Autodesk Inventor part; units mm, degrees
(part 2 of 2)
sketch "Sketch20" plane through (6.35, 0, 0) normal (1, 0, 0) x (0, 0, -1)
  line L0 (-19.4443, 227.7716) -> (-198.6709, 407.7544) construction
  line L1 (-19.4443, 227.7716) -> (0, 0) construction
  circle A0 centre (-198.6709, 407.7544) radius 14.2875
  circle A1 centre (-198.6709, 407.7544) radius 25.4 construction
  arc A2 (-180.6726, 425.6771) -> (-216.6692, 389.8318) centre (-198.6709, 407.7544) ccw
  circle A3 centre (0, 0) radius 14.2875 projected
  arc A4 (-50.2264, 149.2557) -> (-54.8964, 147.6019) centre (0, 0) ccw projected
  arc A5 (-59.2639, 135.1204) -> (-53.6386, 137.4505) centre (-57.3822, 138.5329) ccw projected
  arc A6 (-65.5527, 143.188) -> (-70.0243, 141.0551) centre (0, 0) ccw projected
  arc A7 (-73.0632, 128.1854) -> (-67.7123, 131.0907) centre (-71.5485, 131.776) ccw projected
  arc A8 (-80.1608, 135.5514) -> (-84.385, 132.9629) centre (0, 0) ccw projected
  arc A9 (-86.062, 119.846) -> (-81.044, 123.2948) centre (-84.9309, 123.5752) ccw projected
  arc A10 (-93.8907, 126.4298) -> (-97.8211, 123.4139) centre (0, 0) ccw projected
  arc A11 (-98.1178, 110.1936) -> (-93.4879, 114.1479) centre (-97.3828, 114.0206) ccw projected
  arc A12 (-106.5918, 115.9229) -> (-110.1855, 112.5127) centre (0, 0) ccw projected
  arc A13 (-109.0987, 99.3338) -> (-104.9075, 103.7505) centre (-108.7677, 103.2167) ccw projected
  arc A14 (-118.1252, 104.146) -> (-121.3427, 100.3788) centre (0, 0) ccw projected
  arc A15 (-118.8843, 87.3857) -> (-115.1776, 92.2163) centre (-118.9609, 91.2819) ccw projected
  arc A16 (-128.3643, 91.2281) -> (-131.1704, 87.1452) centre (0, 0) ccw projected
  arc A17 (-127.3673, 74.4802) -> (-124.1859, 79.6718) centre (-127.8508, 78.3471) ccw projected
  arc A18 (-137.197, 77.3106) -> (-139.561, 72.9568) centre (0, 0) ccw projected
  arc A19 (-134.4549, 60.7587) -> (-131.8336, 66.2544) centre (-135.3399, 64.5538) ccw projected
  arc A20 (-144.5266, 62.5461) -> (-146.4225, 57.969) centre (0, 0) ccw projected
  arc A21 (-140.0693, 46.3715) -> (-138.0368, 52.1111) centre (-141.3462, 50.0533) ccw projected
  arc A22 (-150.2727, 47.0963) -> (-151.6798, 42.3461) centre (0, 0) ccw projected
  arc A23 (-144.1492, 31.4762) -> (-142.7278, 37.3968) centre (-145.8039, 35.0044) ccw projected
  arc A24 (-154.3724, 31.1305) -> (-155.2752, 26.2593) centre (0, 0) ccw projected
  arc A25 (-146.6497, 16.2361) -> (-145.8549, 22.2728) centre (-148.6641, 19.572) ccw projected
  arc A26 (7.613, -24.2323) -> (25.308, 2.1605) centre (0, 0) ccw projected
  arc A27 (-156.7808, 14.8237) -> (-157.1695, 9.8848) centre (0, 0) ccw projected
  arc A28 (-147.5434, 0.8181) -> (-147.384, 6.9048) centre (-149.8956, 3.9252) ccw projected
  arc A29 (-157.4714, -1.6456) -> (-157.3417, -6.5981) centre (0, 0) ccw projected
  arc A30 (-146.8207, -14.6089) -> (-147.2984, -8.5388) centre (-149.4847, -11.7647) ccw projected
  arc A31 (-156.4367, -18.0968) -> (-155.7901, -23.0086) centre (0, 0) ccw projected
  arc A32 (-144.4893, -29.8758) -> (-145.5989, -23.8889) centre (-147.4361, -27.3257) ccw projected
  arc A33 (-153.6881, -34.3498) -> (-152.5316, -39.1671) centre (0, 0) ccw projected
  arc A34 (-140.575, -44.8154) -> (-142.3043, -38.9773) centre (-143.7721, -42.5872) ccw projected
  arc A35 (-149.2557, -50.2264) -> (-147.6019, -54.8964) centre (0, 0) ccw projected
  arc A36 (-135.1204, -59.2639) -> (-137.4505, -53.6386) centre (-138.5329, -57.3822) ccw projected
  arc A37 (-143.188, -65.5527) -> (-141.0551, -70.0243) centre (0, 0) ccw projected
  arc A38 (-130.9051, -67.7501) -> (-131.0907, -67.7123) centre (-131.776, -71.5485) ccw projected
  line L2 (-130.9051, -67.7501) -> (7.613, -24.2323) projected
  arc A39 (-44.8154, 140.575) -> (-38.9773, 142.3043) centre (-42.5872, 143.7721) ccw projected
  circle A40 centre (-19.4443, 227.7716) radius 14.2875 projected
  line L3 (25.308, 2.1605) -> (5.8637, 229.932) projected
  arc A41 (5.8637, 229.932) -> (-44.787, 226.0661) centre (-19.4443, 227.7716) ccw projected
  line L4 (-44.787, 226.0661) -> (-39.3751, 145.6486) projected
  line L5 (5.8637, 229.932) -> (-44.7522, 225.6111)
  line L6 (5.8637, 229.932) -> (25.308, 2.1605) projected
  line L7 (-39.3751, 145.6486) -> (-44.787, 226.0661) projected
  line L8 (-216.6692, 389.8318) -> (-44.1488, 216.5834)
  line L9 (-180.6726, 425.6771) -> (-1.446, 245.6942)
  arc A42 (5.8637, 229.932) -> (-44.787, 226.0661) centre (-19.4443, 227.7716) ccw projected
  point P0 (-44.1488, 216.5834)
  dimension "d130" = 254
  dimension "d131" = 140
  dimension "d132" = 28.575
  dimension "d133" = 50.8
  dimension "d156" = 0
  constraints: 10 end point, 6 point on circle, 3 centre point, 3 coincident, 3 tangent, 1 concentric, 1 midpoint, 1 point on line, 35 other
  measures "d130" distance of L0.start L0.end
  measures "d131" angle of L1 L0
  measures "d132" diameter of A0
  measures "d133" diameter of A1
  measures "d156" angle of L8 L9
extrude "Extrusion21" add sketch "Sketch20" against normal blind 6.35 contours L9 A41 L4 L8 A2
sketch "Sketch21" plane through (6.35, 0, 0) normal (1, 0, 0) x (0, 0, -1)
  circle A0 centre (0, 0) radius 146.05
  circle A1 centre (0, 0) radius 97.155
  circle A2 centre (0, 0) radius 80.01
  line L0 (0, 0) -> (-128.3643, 91.2281)
  line L1 (0, 0) -> (0, -146.05)
  line L2 (0, 0) -> (-154.3724, 31.1305)
  arc A3 (-127.3673, 74.4802) -> (-124.1859, 79.6718) centre (-127.8508, 78.3471) ccw projected
  point P0 (0, -97.155)
  point P1 (0, -80.01)
  point P2 (-65.2173, 46.3497)
  point P3 (-79.1925, 56.2818)
  point P4 (-78.4311, 15.8163)
  point P5 (-95.2378, 19.2055)
  dimension "d137" = 292.1
  dimension "d138" = 48.895
  dimension "d139" = 17.145
  constraints: 6 end point, 3 coincident, 2 centre point, 1 vertical, 1 vertical alignment, 2 other
  measures "d139" radial gap between concentric circles of A1 A2
extrude "Extrusion22" cut sketch "Sketch21" against normal blind 6.35 contours A1 L2 A2 L1 | A1 L0 A2 L2
fillet "Fillet2" radius 8.5725 2 edges at (3.175, 56.2818, 79.1925) (3.175, 46.3497, 65.2173)
fillet "Fillet3" radius 6.35 2 edges at (3.175, -52.3392, 81.8517) (3.175, -46.9727, 64.7701)
sketch "Sketch22" plane through (0, 0, 0) normal (-1, 0, 0) x (0, 0, 1)
  circle A0 centre (19.4443, 227.7716) radius 14.2875 projected
  circle A1 centre (19.4443, 227.7716) radius 25.4
  circle A2 centre (198.6709, 407.7544) radius 14.2875 projected
  circle A3 centre (198.6709, 407.7544) radius 25.4
  arc A4 (216.6692, 389.8318) -> (44.7712, 225.8313) centre (235.9913, 209.2855) ccw projected
  line L0 (216.6692, 389.8318) -> (37.4426, 209.8489)
  arc A5 (60.2698, -45.5588) -> (67.5328, -42.906) centre (62.173, -39.5007) ccw projected
  arc A6 (67.5328, -42.906) -> (69.3967, 39.8208) centre (0, 0) ccw projected
  arc A7 (85.7456, -45.6814) -> (84.2674, 48.3539) centre (0, 0) ccw projected
  arc A8 (85.7456, -45.6814) -> (89.4466, -54.7252) centre (91.3498, -48.6671) ccw projected
  line L1 (89.4466, -54.7252) -> (130.9051, -67.7501) projected
  arc A9 (131.0907, -67.7123) -> (130.9051, -67.7501) centre (131.776, -71.5485) ccw projected
  arc A10 (141.0551, -70.0243) -> (143.188, -65.5527) centre (0, 0) ccw projected
  arc A11 (137.4505, -53.6386) -> (135.1204, -59.2639) centre (138.5329, -57.3822) ccw projected
  arc A12 (147.6019, -54.8964) -> (149.2557, -50.2264) centre (0, 0) ccw projected
  arc A13 (142.3043, -38.9773) -> (140.575, -44.8154) centre (143.7721, -42.5872) ccw projected
  arc A14 (152.5316, -39.1671) -> (153.6881, -34.3498) centre (0, 0) ccw projected
  arc A15 (145.5989, -23.8889) -> (144.4893, -29.8758) centre (147.4361, -27.3257) ccw projected
  arc A16 (155.7901, -23.0086) -> (156.4367, -18.0968) centre (0, 0) ccw projected
  arc A17 (147.2984, -8.5388) -> (146.8207, -14.6089) centre (149.4847, -11.7647) ccw projected
  arc A18 (157.3417, -6.5981) -> (157.4714, -1.6456) centre (0, 0) ccw projected
  arc A19 (147.384, 6.9048) -> (147.5434, 0.8181) centre (149.8956, 3.9252) ccw projected
  arc A20 (157.1695, 9.8848) -> (156.7808, 14.8237) centre (0, 0) ccw projected
  arc A21 (145.8549, 22.2728) -> (146.6497, 16.2361) centre (148.6641, 19.572) ccw projected
  arc A22 (155.2752, 26.2593) -> (154.3724, 31.1305) centre (0, 0) ccw projected
  arc A23 (142.7278, 37.3968) -> (144.1492, 31.4762) centre (145.8039, 35.0044) ccw projected
  arc A24 (151.6798, 42.3461) -> (150.2727, 47.0963) centre (0, 0) ccw projected
  arc A25 (138.0368, 52.1111) -> (140.0693, 46.3715) centre (141.3462, 50.0533) ccw projected
  arc A26 (146.4225, 57.969) -> (144.5266, 62.5461) centre (0, 0) ccw projected
  arc A27 (131.8336, 66.2544) -> (134.4549, 60.7587) centre (135.3399, 64.5538) ccw projected
  arc A28 (139.561, 72.9568) -> (137.197, 77.3106) centre (0, 0) ccw projected
  arc A29 (124.1859, 79.6718) -> (127.3673, 74.4802) centre (127.8508, 78.3471) ccw projected
  arc A30 (131.1704, 87.1452) -> (128.3643, 91.2281) centre (0, 0) ccw projected
  arc A31 (115.1776, 92.2163) -> (118.8843, 87.3857) centre (118.9609, 91.2819) ccw projected
  arc A32 (121.3427, 100.3788) -> (118.1252, 104.146) centre (0, 0) ccw projected
  arc A33 (104.9075, 103.7505) -> (109.0987, 99.3338) centre (108.7677, 103.2167) ccw projected
  arc A34 (110.1855, 112.5127) -> (106.5918, 115.9229) centre (0, 0) ccw projected
  arc A35 (93.4879, 114.1479) -> (98.1178, 110.1936) centre (97.3828, 114.0206) ccw projected
  arc A36 (97.8211, 123.4139) -> (93.8907, 126.4298) centre (0, 0) ccw projected
  arc A37 (81.044, 123.2948) -> (86.062, 119.846) centre (84.9309, 123.5752) ccw projected
  arc A38 (84.385, 132.9629) -> (80.1608, 135.5514) centre (0, 0) ccw projected
  arc A39 (67.7123, 131.0907) -> (73.0632, 128.1854) centre (71.5485, 131.776) ccw projected
  arc A40 (70.0243, 141.0551) -> (65.5527, 143.188) centre (0, 0) ccw projected
  arc A41 (53.6386, 137.4505) -> (59.2639, 135.1204) centre (57.3822, 138.5329) ccw projected
  arc A42 (54.8964, 147.6019) -> (50.2264, 149.2557) centre (0, 0) ccw projected
  arc A43 (38.9773, 142.3043) -> (44.8154, 140.575) centre (42.5872, 143.7721) ccw projected
  line L2 (39.3751, 145.6486) -> (44.1488, 216.5834) projected
  line L3 (-5.8637, 229.932) -> (-25.308, 2.1605) projected
  arc A44 (-25.308, 2.1605) -> (-7.613, -24.2323) centre (0, 0) ccw projected
  line L4 (-7.613, -24.2323) -> (60.2698, -45.5588) projected
  circle A45 centre (0, 0) radius 14.2875 projected
  circle A46 centre (19.4443, 227.7716) radius 14.2875 projected
  arc A47 (1.446, 245.6942) -> (-5.8637, 229.932) centre (19.4443, 227.7716) ccw projected
  line L5 (44.1488, 216.5834) -> (216.6692, 389.8318) projected
  arc A48 (216.6692, 389.8318) -> (180.6726, 425.6771) centre (198.6709, 407.7544) ccw projected
  line L6 (180.6726, 425.6771) -> (1.446, 245.6942) projected
  arc A49 (84.2674, 48.3539) -> (69.3967, 39.8208) centre (76.8321, 44.0874) ccw projected
  point P0 (44.7712, 225.8313)
  point P1 (44.1488, 216.5834)
  dimension "d147" = 50.8
  dimension "d148" = 50.8
  constraints: 2 coincident, 2 end point, 1 centre point, 1 point on circle, 1 tangent, 40 other
  measures "d148" diameter of A3
extrude "Extrusion23" [suppressed]
fillet "Fillet4" [suppressed]
fillet "Fillet5" radius 101.6 1 edges at (3.175, 216.5834, 44.1488)
sketch "Sketch23" plane through (6.35, 0, 0) normal (1, 0, 0) x (0, 0, -1)
  line L0 (0, 0) -> (-4.321, 50.6159)
  line L1 (25.308, 2.1605) -> (5.8637, 229.932) projected
  circle A0 centre (-4.321, 50.6159) radius 3.2512
  dimension "d157" = 50.8
  dimension "d158" = 6.5024
  constraints: 2 end point, 1 centre point, 1 coincident, 1 parallel
  measures "d157" distance of L0.start L0.end
  measures "d158" diameter of A0
extrude "Extrusion24" cut sketch "Sketch23" against normal blind 6.35
equation "\"PD\" = 304.8"
equation "\"a\" = 14.5deg"
equation "\"add\" = mod"
equation "\"ded\" = 6.35"
equation "\"RD\" = PD - 2 * ded"
equation "\"OD\" = PD + 2 * add"
equation "\"mod\" = 5.08"
body "Solid2"
